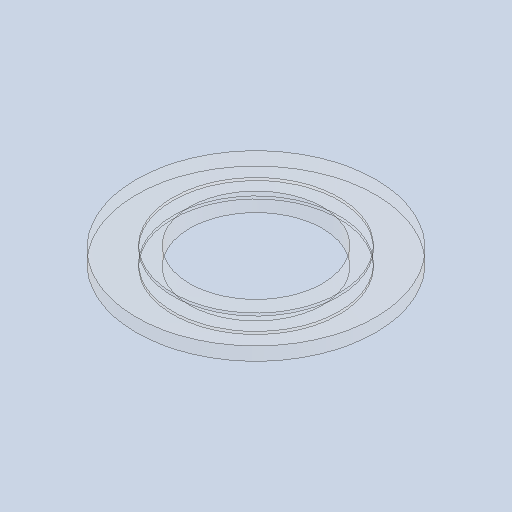
# Autodesk Inventor part: Apoio Contato
Saved by Autodesk Inventor 2022.2 (Build 262287000, 287)
## iProperties
Created: 2021-01-23
Part Number: Apoio Contato
Material: Plástico SAN
Document SubType Name: Modeling
Designer: João
Density: 1.068 g/cm^3
Appearance: Policarbonato - Transparente
Mass: 0.000206765 g
Surface Area: 0.0468097 cm^2
Volume: 0.000193601 cm^3
Author: João
Autodesk Inventor part; units mm, degrees
ref_plane "YZ Plane" through (0, 0, 0) normal (1, 0, 0) x (0, 1, 0)
ref_plane "XZ Plane" through (0, 0, 0) normal (0, 1, 0) x (-1, 0, 0)
ref_plane "XY Plane" through (0, 0, 0) normal (0, 0, 1) x (1, 0, 0)
sketch "Esboço1" plane through (0, 0, 0) normal (0, 1, 0) x (-1, 0, 0)
  circle A0 centre (0, 0) radius 0.9
  circle A1 centre (0, 0) radius 0.5
  dimension "d0" = 1.8
  dimension "d1" = 1
  constraints: 2 centre point, 2 coincident
  measures "d0" diameter of A0
  measures "d1" diameter of A1
extrude "Extrusão1" add sketch "Esboço1" along normal blind 0.1
sketch "Esboço2" plane through (0, 0.1, 0) normal (0, 1, 0) x (1, 0, 0)
  circle A0 centre (0, 0) radius 0.625
  circle A1 centre (0, 0) radius 0.5 projected
  dimension "d4" = 1.25
  constraints: 1 centre point, 1 coincident
  measures "d4" diameter of A0
extrude "Extrusão2" add sketch "Esboço2" along normal blind 0.02 and the other way blind 0.12
